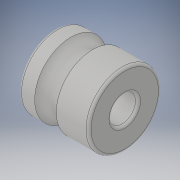
# Autodesk Inventor part: 040400DR-22-H4W(0.5)3_ir
Saved by Autodesk Inventor 2024 (Build 280153000, 153)
## iProperties
Created: 2023-06-17
Part Number: 040400DR-22-H4W(0.5)3_ir
Material: Generic
Catalog Web Link: www.cadenas.de
Description: DR-H ir-D-Series bearings
Vendor: TOKBEARING
Document SubType Name: Modeling
Designer: psAdmin
Manufacturer: TOKBEARING
Mass: 8300 g
Surface Area: 6.48185 cm^2
Volume: 0.781937 cm^3
Density: 1 g/cm^3
Appearance: PSOLRGB-175-175-175
Category: PARTsolutions
Company: TOKBEARING
PSOL_IDENT_0: {$CADENAS_DATA/23d-libs/tok_bearing/d_series_bearings/dr_h/dr_h_ir.prj},191 {VTYP=3D},{NB=040400DR-2
PSOL_IDENT_1: 2-H4W(0.5)3_ir},{LINA=040400DR-22-H4W(0.5)3_ir},{NN=DR-H ir},{DATE=16.12.2020 00:38:04},{GEOMDATE=19
PSOL_IDENT_2: .02.2013 00:00:00},{VERSION=},{LINEID=1750},{WBVAR=},{WBNUMERIC=}  {NB=040400DR-22-H4W(0.5)3_ir},{LI
PSOL_IDENT_3: NA=040400DR-22-H4W(0.5)3_ir},{KT=DUMMY},{IDNR=},{CODE=040400},{PN=DR-22-H4W(0.5)3},{D=22},{SD=4.0},{
PSOL_IDENT_4: W=7.0},{W1=0.5},{W1X=0.500},{W2=3},{W2X=3.000},{LOAD=196 (20)},{TYPE=12},{QTY=1.000},{GW=8.3},{BD=3.
PSOL_IDENT_5: 78},{OP=40.2862},{N=5},{R=6.415},{GP=3.64}
NB: 040400DR-22-H4W(0.5)3_ir
NN: DR-H ir
NT: D-Series bearings
NBSYN: $CODE.$PN._ir
LINA: 040400DR-22-H4W(0.5)3_ir
CATALOG: TOK, Inc
CODE: 040400
PN: DR-22-H4W(0.5)3
D: 22
SD: 4
W: 7
W1: 0.5
W2: 3
LOAD: 196 (20)
TYPE: 12
QTY: 1.000
GW: 8.3
SUPPLIER: TOKBEARING
ARTICLENO: 040400DR-22-H4W(0.5)3_ir
BOMINFO: 040400DR-22-H4W(0.5)3_ir
CREATOR: CADENAS GmbH
Title: 040400DR-22-H4W(0.5)3_ir
Author: Cadenas PARTsolutions
Comments: D-Series bearings
Autodesk Inventor part; units mm, degrees
sketch "Sketch_4" plane through (0, 0, 0) normal (0, 0, 1) x (1, 0, 0)
  line L0 (10.5, 0) -> (0, 0)
  arc A0 (0, 2.3889) -> (0.3889, 2) centre (0.3889, 2.3889) ccw
  line L1 (0.3889, 2) -> (10.1111, 2)
  arc A1 (10.1111, 2) -> (10.5, 2.3889) centre (10.1111, 2.3889) ccw
  line L2 (10.5, 2.3889) -> (10.5, 5.0811)
  arc A2 (10.5, 5.0811) -> (10.1111, 5.47) centre (10.1111, 5.0811) ccw
  line L3 (10.1111, 5.47) -> (5.6368, 5.47)
  arc A3 (2.3632, 5.47) -> (5.6368, 5.47) centre (4, 6.415) ccw
  line L4 (2.3632, 5.47) -> (0.3889, 5.47)
  arc A4 (0.3889, 5.47) -> (0, 5.0811) centre (0.3889, 5.0811) ccw
  line L5 (0, 5.0811) -> (0, 2.3889)
  constraints: 12 end point, 10 point on circle, 5 centre point
revolve "Revolution1" add sketch "Sketch_4" angle 360 about axis through (10.5, 0, 0) along (1, 0, 0)
ref_plane "Dummy_IR_XY" through (0, 0, 0) normal (1, 0, 0) x (0, 0, -1)
ref_plane "Dummy_IR_YZ" through (0, 0, 0) normal (0, 0, -1) x (0, 1, 0)
ref_plane "Dummy_IR_ZX" through (0, 0, 0) normal (0, 1, 0) x (1, 0, 0)
ref_plane "IR_OR_XY" through (0, 0, 0) normal (1, 0, 0) x (0, 0, -1)
ref_plane "IR_OR_YZ" through (0, 0, 0) normal (0, 0, -1) x (0, 1, 0)
ref_plane "IR_OR_ZX" through (0, 0, 0) normal (0, 1, 0) x (1, 0, 0)
body "Solid1"
